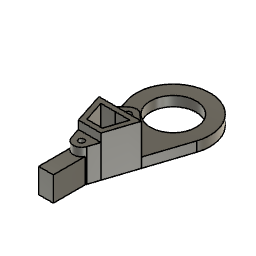
lower_upper v1 (Autodesk Fusion 360 design; units mm, degrees)
Autodesk Fusion 360 part; units mm, degrees
sketch "Sketch1" plane through (0, 0, 0) normal (0, 0, 1) x (1, 0, 0)
  line L0 (-4.5, 9.5706) -> (-4.4999, -10)
  line L1 (-4.4999, -10) -> (4.5001, -10)
  line L2 (4.5001, -10) -> (4.5, 9.5706)
  line L3 (0.0001, -10) -> (0, 51) construction
  line L4 (0, 51) -> (0, 67.95) construction
  line L5 (0, 10) -> (0, 11.75)
  circle A0 centre (0, 67.95) radius 14
  circle A1 centre (0, 11.75) radius 1.75
  line L6 (0.0001, 13.5) -> (0.0001, 16.7501) construction
  line L7 (0.0001, 13.72) -> (0, 38.45) construction
  line L8 (0, 38.45) -> (0, 40.45) construction
  circle A2 centre (0, 40.45) radius 1.75
  line L9 (0, 11.75) -> (0, 46.87) construction
  line L10 (21.3814, 60.9438) -> (4.7514, 10.1931)
  line L11 (8.8876, 32.45) -> (4.7365, 19.7818)
  line L12 (0, 32.45) -> (8.8876, 32.45)
  line L13 (4.7365, 19.7818) -> (0.0001, 19.7818)
  line L14 (0, 35.45) -> (13.0276, 35.45)
  line L15 (0.0001, 16.7501) -> (6.9, 16.7501)
  line L16 (0, 32.45) -> (-8.8876, 32.45)
  line L17 (-8.8876, 32.45) -> (-4.7364, 19.7818)
  line L18 (-4.7364, 19.7818) -> (0.0001, 19.7818)
  line L19 (0.0001, 16.7501) -> (-6.8999, 16.7501)
  line L20 (-21.3813, 60.9437) -> (-4.7513, 10.1931)
  line L21 (0, 35.45) -> (-13.0275, 35.45)
  arc A3 (-4.7617, 10.2248) -> (4.7514, 10.1931) centre (0, 11.75) ccw
  line L22 (13.0276, 35.45) -> (3.3453, 44.1661)
  line L23 (-13.0275, 35.45) -> (-3.3452, 44.1661)
  arc A4 (3.3453, 44.1661) -> (-3.3452, 44.1661) centre (0, 40.45) ccw
  arc A5 (0, 35.45) -> (0, 35.45) centre (0, 40.45) ccw
  arc A6 (0, 45.45) -> (0, 45.45) centre (0, 67.95) ccw
  arc A7 (21.3814, 60.9438) -> (-21.3813, 60.9437) centre (0, 67.95) ccw
  dimension "d1" = 9
  dimension "d6" = 28
  dimension "d7" = 45
  dimension "d8" = 3.5
  dimension "d15" = 3.5
  dimension "d27" = 10
  dimension "d28" = 20
  dimension "d36" = 10
  constraint parallel L0 L2
  constraint midpoint L1 L3.start
  constraint perpendicular L1 L3
  constraint parallel L3 L4
  constraint vertical L5
  constraint coincident L4.end A0.centre
  constraint concentric A0 A6
  constraint coincident L5.end A1.centre
  constraint coincident A1 L6.start
  constraint coincident L3 L6.start
  constraint parallel L3 L6
  constraint parallel L3 L7
  constraint coincident L8.end A2.centre
  constraint parallel L3 L9
  constraint coincident L5.start A1
  constraint coincident L0.start A3
  constraint coincident L2.end A3
  constraint concentric A2 A4
  constraint tangent A4 A6
  constraint coincident L10.start A6
  constraint tangent L10 A6
  constraint tangent L10 A3
  constraint horizontal L13
  constraint coincident L7 L13.end
  constraint coincident L3 L13.end
  constraint horizontal L14
  constraint coincident L7 L14.start
  constraint coincident L10 L14.end
  constraint tangent L14 A4
  constraint coincident L10 L15.end
  constraint perpendicular L7 L15
  constraint symmetric L3 L6.end L15.start
  constraint symmetric L3 L10.start L20.start
  constraint symmetric L3 L10.end L20.end
  constraint symmetric L3 L12.start L16.start
  constraint symmetric L3 L11.start L16.end
  constraint symmetric L3 L11.end L17.end
  constraint symmetric L3 L13.end L18.end
  constraint symmetric L3 L14.start L21.start
  constraint symmetric L3 L14.end L21.end
  constraint symmetric L3 L15.end L19.end
  constraint coincident L20 A3.start
  constraint tangent L22 A4
  constraint tangent L23 A4
  constraint coincident L9 L14.start
  constraint concentric A4 A5
  constraint coincident L3 A6.start
  constraint concentric A6 A7
  measures "d1" distance of L0.end L1.end
  measures "d6" diameter of A0
  measures "d7" diameter of A6
  measures "d8" diameter of A1
  measures "d15" diameter of A2
  measures "d27" diameter of A3
  measures "d28" distance of L3.start L5.start
  measures "d36" diameter of A4
extrude "Extrude1" add sketch "Sketch1" along normal blind 6 contours L20 L23 A4 A5 A6 | L10 L22 A4 A5 A6 | A6 A7 makes body 1
extrude "Extrude2" add sketch "Sketch1" along normal blind 15 separate body contours L0 L1 L2 A3 makes body 2
extrude "Extrude3" add sketch "Sketch1" along normal blind 20 contours L10 L15 L19 L20 A3 | L21 L23 A5 | L14 L22 A5 | A4 A5 bodies 1 2
extrude "Extrude5" add sketch "Sketch1" along normal blind 25 separate body contours L10 L14 L15 L19 L20 L21 makes body 3
